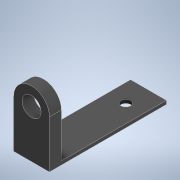
# Autodesk Inventor part: Half Bearing Block
Saved by Autodesk Inventor 2022 (Build 260153000, 153)
## iProperties
Created: 2021-12-04
Part Number: Half Bearing Block
Material: Generic
Document SubType Name: Modeling
Designer: LEGION SMIT
Density: 1 g/cm^3
Appearance: Generic
Author: LEGION SMIT
Autodesk Inventor part; units mm, degrees
ref_plane "YZ Plane" through (0, 0, 0) normal (1, 0, 0) x (0, 1, 0)
ref_plane "XZ Plane" through (0, 0, 0) normal (0, 1, 0) x (-1, 0, 0)
ref_plane "XY Plane" through (0, 0, 0) normal (0, 0, 1) x (1, 0, 0)
sketch "Sketch1" plane through (0, 0, 0) normal (0, 0, 1) x (1, 0, 0)
  circle A0 centre (0, 0) radius 4
  arc A1 (7.5, 0) -> (-7.5, 0) centre (0, 0) ccw
  line L0 (-7.5, 0) -> (7.5, 0)
  line L1 (7.5, 0) -> (7.5, -20)
  line L2 (7.5, -20) -> (-7.5, -20)
  line L3 (-7.5, -20) -> (-7.5, 0)
  dimension "d0" = 8
  dimension "d1" = 15
  dimension "d2" = 15
  dimension "d3" = 20
  constraints: 8 end point, 2 centre point, 2 coincident, 2 parallel, 2 point on circle, 1 horizontal, 1 perpendicular
  measures "d0" diameter of A0
  measures "d1" diameter of A1
  measures "d2" distance of L1.end L2.end
  measures "d3" distance of L0.end L1.end
extrude "Extrusion1" add sketch "Sketch1" along normal mid plane 5 contours L0 L1 L2 L3 A0 | A0 L0 A1
sketch "Sketch2" plane through (0, 0, -2.5) normal (0, 0, -1) x (-1, 0, 0)
  line L0 (7.5, -20) -> (-7.5, -20) projected
  line L1 (-7.5, -20) -> (7.5, -20)
  line L2 (7.5, -20) -> (7.5, -18.5)
  line L3 (7.5, -18.5) -> (-7.5, -18.5)
  line L4 (-7.5, -18.5) -> (-7.5, -20)
  point P0 (0, 0)
  dimension "d6" = 15
  dimension "d7" = 1.5
  constraints: 8 end point, 2 parallel, 1 horizontal, 1 perpendicular
  measures "d6" distance of L3.end L2.end
  measures "d7" distance of L2.end L1.end
extrude "Extrusion2" add sketch "Sketch2" along normal blind 44
sketch "Sketch3" plane through (-7.5, -18.5, -2.5) normal (0, 1, 0) x (1, 0, 0)
  line L0 (0, -5) -> (15, -5) projected
  line L1 (7.5, -5) -> (7.5, 4.5)
  line L2 (7.5, 4.5) -> (7.5, 34.5)
  point P0 (7.5, -2.5)
  dimension "d10" = 9.5
  dimension "d11" = 30
  constraints: 4 end point, 2 vertical, 1 midpoint
  measures "d10" distance of L1.start L1.end
  measures "d11" distance of L1.end L2.end
hole "Hole1" at (0, -18.5, -7) at (0, -18.5, -37) direction (0, -1, 0) diameter 4 depth 6
body "Solid1"
